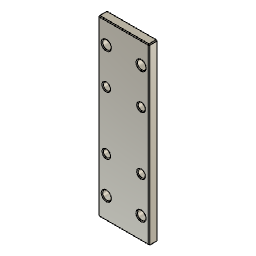
Y motor reinforcement plate (Autodesk Fusion 360 design; units mm, degrees)
Autodesk Fusion 360 part; units mm, degrees
sketch "Sketch1" plane through (0, 0, 0) normal (0, 1, 0) x (1, 0, 0)
  line L0 (17.5, -60) -> (-17.5, -60)
  line L1 (-17.5, -60) -> (-17.5, 60)
  line L2 (-17.5, 60) -> (17.5, 60)
  line L3 (17.5, 60) -> (17.5, -60)
  line L4 (17.5, -60) -> (-17.5, 60) construction
  line L5 (-17.5, -60) -> (17.5, 60) construction
  line L6 (12, -60) -> (12, 60) construction
  line L7 (-12, -60) -> (-12, 60) construction
  line L8 (-17.5, -20) -> (17.5, -20) construction
  line L9 (-17.5, -45) -> (17.5, -45) construction
  line L10 (-17.5, 20) -> (17.5, 20) construction
  line L11 (-17.5, 45) -> (17.5, 45) construction
  circle A0 centre (-12, -45) radius 3
  circle A1 centre (12, -45) radius 3
  circle A2 centre (-12, -20) radius 2.5
  circle A3 centre (12, -20) radius 2.5
  circle A4 centre (-12, 20) radius 2.5
  circle A5 centre (12, 20) radius 2.5
  circle A6 centre (-12, 45) radius 3
  circle A7 centre (12, 45) radius 3
  dimension "d1" = 120
  dimension "d2" = 35
  dimension "d3" = 5.5
  dimension "d4" = 5.5
  dimension "d5" = 24
  dimension "d6" = 40
  dimension "d7" = 25
  dimension "d8" = 25
  dimension "d9" = 20
  dimension "d10" = 6
  dimension "d11" = 6
  dimension "d12" = 5
  dimension "d13" = 5
  dimension "d14" = 5
  dimension "d15" = 5
  dimension "d16" = 6
  dimension "d17" = 6
  constraint perpendicular L0 L1
  constraint parallel L0 L2
  constraint parallel L1 L3
  constraint horizontal L0
  constraint coincident L4 origin
  constraint coincident L5 origin
  constraint coincident L0 L6.start
  constraint coincident L2 L6.end
  constraint perpendicular L2 L6
  constraint coincident L2 L7.end
  constraint perpendicular L2 L7
  constraint coincident L1 L8.start
  constraint coincident L3 L8.end
  constraint perpendicular L3 L8
  constraint coincident L1 L9.start
  constraint coincident L3 L9.end
  constraint perpendicular L3 L9
  constraint coincident L1 L10.start
  constraint perpendicular L6 L10
  constraint coincident L1 L11.start
  constraint perpendicular L6 L11
  constraint coincident L7 A0.centre
  constraint coincident L9 A0.centre
  constraint coincident L9 A1.centre
  constraint coincident L6 A1.centre
  constraint coincident L7 A2.centre
  constraint coincident L8 A2.centre
  constraint coincident L8 A3.centre
  constraint coincident L6 A3.centre
  constraint coincident L10 A4.centre
  constraint coincident L7 A4.centre
  constraint coincident L10 A5.centre
  constraint coincident L6 A5.centre
  constraint coincident L7 A6.centre
  constraint coincident L11 A6.centre
  constraint coincident L6 A7.centre
  constraint coincident L11 A7.centre
  measures "d1" distance of L0.end L1.end
  measures "d2" distance of L1.end L2.end
  measures "d3" distance of L1 L7
  measures "d4" distance of L3 L6
  measures "d5" distance of L6 L7
  measures "d6" distance of L8 L10
  measures "d7" distance of L8 L9
  measures "d8" distance of L10 L11
  measures "d9" distance of origin L8 L0.start
  measures "d10" diameter of A0
  measures "d11" diameter of A1
  measures "d12" diameter of A2 L0.start
  measures "d13" diameter of A3 L0.start
  measures "d14" diameter of A4
  measures "d15" diameter of A5
  measures "d16" diameter of A6
  measures "d17" diameter of A7
extrude "Extrude1" add sketch "Sketch1" along normal blind 6
chamfer "Chamfer1" distance 0.5 angle 45 27 edges at (0, 0, 60) (-17.5, 3, 60) (0, 6, 60) (17.5, 3, 60) (17.5, 6, 0) (17.5, 0, 0) (-17.5, 0, 0) (-14.797, 0, 43.9152) (9.203, 0, 43.9152) (-14.3308, 0, 19.096) (9.6692, 0, 19.096) (9.6692, 0, -20.904) (-14.3308, 0, -20.904) (-14.797, 0, -46.0848) (9.203, 0, -46.0848) (0, 0, -60) (9.203, 6, -46.0848) (0, 6, -60) (-17.5, 3, -60) (-17.5, 6, 0) (-14.797, 6, -46.0848) (-14.3308, 6, -20.904) (9.6692, 6, -20.904) (9.6692, 6, 19.096) (-14.3308, 6, 19.096) (-14.797, 6, 43.9152) (9.203, 6, 43.9152)
named bodies: "Plate"
